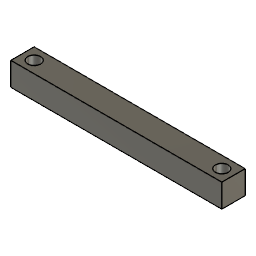
Spiegelhouder deel 2 (Autodesk Fusion 360 design; units mm, degrees)
part number: 2026-06-04-17-11-57-773
Autodesk Fusion 360 part; units mm, degrees
sketch "Sketch1" plane through (0, 0, 0) normal (0, 0, 1) x (1, 0, 0)
  line L0 (-45, -5) -> (45, -5)
  line L1 (45, -5) -> (45, 5)
  line L2 (45, 5) -> (-45, 5)
  line L3 (-45, 5) -> (-45, -5)
  line L4 (-45, -5) -> (45, 5) construction
  line L5 (45, -5) -> (-45, 5) construction
  dimension "d1" = 90
  dimension "d2" = 10
  constraint horizontal L0
  constraint perpendicular L0 L1
  constraint parallel L0 L2
  constraint parallel L1 L3
  constraint coincident L4 origin
  constraint coincident L5 origin
  measures "d1" distance of L1.end L2.end
  measures "d2" distance of L0.end L1.end
extrude "Extrude1" add sketch "Sketch1" along normal blind 10
sketch "Sketch2" plane through (0, 0, 10) normal (0, 0, 1) x (-1, 0, 0)
  line L0 (45, -5) -> (45, 5)
  line L1 (45, 5) -> (-45, 5)
  line L2 (-45, 5) -> (-45, -5)
  line L3 (-45, -5) -> (45, -5)
  circle A0 centre (-40, 0) radius 2.75
  circle A1 centre (-40, 0) radius 2.1
  dimension "d5" = 5.5
  dimension "d6" = 4.2
  dimension "d7" = 5
  dimension "d8" = 5
  constraint concentric A0 A1
  measures "d5" diameter of A0
  measures "d6" diameter of A1
  measures "d7" distance of L1 A0.centre
  measures "d8" distance of L2 A0.centre
extrude "Extrude2" cut sketch "Sketch2" against normal blind 10 contours A1
extrude "Extrude3" cut sketch "Sketch2" against normal blind 4 contours A0
mirror "Mirror1" about plane through (0, 0, 0) normal (1, 0, 0) of "Extrude2", "Extrude3"
scale "Scale1" factor 1.008 about (45, 5, 0) bodies 1
